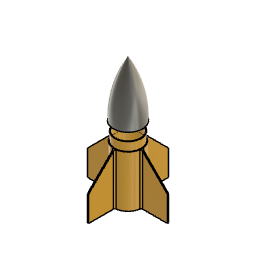
Vlad Rocket 9cone v1 (Autodesk Fusion 360 design; units mm, degrees)
Autodesk Fusion 360 part; units mm, degrees
sketch "Sketch1" plane through (0, 0, 0) normal (0, 0, 1) x (1, 0, 0)
  circle A0 centre (0, 0) radius 12.319
  circle A1 centre (0, 0) radius 11.176
  line L0 (1.016, 25.521) -> (0, 25.521)
  line L1 (-0.508, 25.4) -> (0.508, 25.4)
  line L2 (-0.508, -25.4) -> (-0.508, -12.3085)
  line L3 (0.508, -12.3085) -> (0.508, -25.4)
  line L4 (25.4, 0.508) -> (25.4, -0.508)
  line L5 (0.508, -25.4) -> (-0.508, -25.4)
  line L6 (-25.4, 0.508) -> (-25.4, -0.508)
  line L7 (-0.508, 12.3085) -> (-0.508, 25.4)
  line L8 (0.508, 25.4) -> (0.508, 12.3085)
  line L9 (-25.4, 0.508) -> (-12.3085, 0.508)
  line L10 (-12.3085, -0.508) -> (-25.4, -0.508)
  line L11 (12.3085, 0.508) -> (25.4, 0.508)
  line L12 (25.4, -0.508) -> (12.3085, -0.508)
  dimension "d1" = 24.638
  dimension "d2" = -1.143
  dimension "d8" = 1.016
  constraint coincident A0.centre A1.centre
  constraint horizontal L0
  constraint perpendicular L4 L12
  constraint coincident A0 L7.start
  constraint coincident A0 L8.end
  constraint coincident A0 L9.end
  constraint coincident A0 L10.start
  constraint coincident A0 L12.end
  constraint coincident A0 L11.start
  constraint coincident A0 L3.start
  constraint coincident A0 L2.end
  measures "d1" diameter of A0
  measures "d8" distance of L1.start L1.end
extrude "Extrude1" add sketch "Sketch1" along normal blind 45.72 makes body 1
extrude "Extrude2" add 1 faces at (25.4, 0.1693, 15.24) along direction (1, 0, 0) blind 10.16 on bodies 1 bodies 1
extrude "Extrude3" add 1 faces at (0.1693, -25.4, 15.24) along direction (0, -1, 0) blind 10.16 on bodies 1 bodies 1
extrude "Extrude4" add 1 faces at (-0.1693, 25.4, 15.24) along direction (0, 1, 0) blind 10.16 on bodies 1 bodies 1
extrude "Extrude5" add 1 faces at (-25.4, 0.1693, 15.24) along direction (-1, 0, 0) blind 10.16 on bodies 1 bodies 1
chamfer "Chamfer1" distance 23.241 angle 45 4 edges at (0, 35.56, 45.72) (35.56, 0, 45.72) (0, -35.56, 45.72) (-35.56, 0, 45.72) on bodies 1
sketch "Sketch2" plane through (0, 0, 45.72) normal (0, 0, 1) x (-1, 0, 0)
  line L0 (12.319, -0.508) -> (12.319, 0.508)
  line L1 (12.319, 0.508) -> (12.3085, 0.508)
  arc A0 (12.3085, 0.508) -> (0.508, 12.3085) centre (0, 0) ccw
  line L2 (0.508, 12.3085) -> (0.508, 12.319)
  line L3 (0.508, 12.319) -> (-0.508, 12.319)
  line L4 (-0.508, 12.319) -> (-0.508, 12.3085)
  arc A1 (-0.508, 12.3085) -> (-12.3085, 0.508) centre (0, 0) ccw
  line L5 (-12.3085, 0.508) -> (-12.319, 0.508)
  line L6 (-12.319, 0.508) -> (-12.319, -0.508)
  line L7 (-12.319, -0.508) -> (-12.3085, -0.508)
  arc A2 (-12.3085, -0.508) -> (-0.508, -12.3085) centre (0, 0) ccw
  line L8 (-0.508, -12.3085) -> (-0.508, -12.319)
  line L9 (-0.508, -12.319) -> (0.508, -12.319)
  line L10 (0.508, -12.319) -> (0.508, -12.3085)
  arc A3 (0.508, -12.3085) -> (12.3085, -0.508) centre (0, 0) ccw
  line L11 (12.3085, -0.508) -> (12.319, -0.508)
  circle A4 centre (0, 0) radius 11.176
  circle A5 centre (0, 0) radius 11.176
  circle A6 centre (0, 0) radius 11.7852
  dimension "d22" = 0.6092
  constraint coincident A0.centre A1.centre
extrude "Extrude6" add sketch "Sketch2" along normal blind 7.62 contours A6 bodies 1
fillet "Fillet1" radius 1.27 8 edges at (0.508, -12.3085, 22.86) (12.3085, -0.508, 22.86) (12.3085, 0.508, 22.86) (0.508, 12.3085, 22.86) (-0.508, 12.3085, 22.86) (-12.3085, 0.508, 22.86) (-0.508, -12.3085, 22.86) (-12.3085, -0.508, 22.86) on bodies 1
ref_plane "WorkPlane1" through (24.5161, 0, 22.2834) normal (0, -1, 0) x (1, 0, 0)
sketch "Sketch3" plane through (24.5161, 0, 22.2834) normal (0, -1, 0) x (1, 0, 0)
  arc A0 (-25.4942, 100.8177) -> (-37.7175, 33.3986) centre (183.0643, 28.1876) ccw
  arc A1 (-25.4942, 97.4476) -> (-36.6325, 33.3729) centre (183.0643, 28.1876) ccw
  line L0 (-25.4942, 97.4476) -> (-25.4942, 100.8177)
  line L1 (-36.6325, 33.3729) -> (-37.7175, 33.3986)
  constraint concentric A0 A1
ref_plane "WorkPlane2" through (0, 24.5161, 22.2834) normal (1, 0, 0) x (0, 1, 0)
sketch "Sketch4" plane through (0, 24.5161, 22.2834) normal (1, 0, 0) x (0, 1, 0)
  arc A0 (-10.16, 30.48) -> (-25.4, 88.9) centre (-116.0318, 34.0591) ccw
  line L0 (-12.303, -22.2834) -> (-12.303, 23.4366)
  arc A1 (-11.43, 30.48) -> (-25.4, 87.63) centre (-116.1455, 35.1653) ccw
  line L1 (-10.16, 30.48) -> (-11.43, 30.48)
  line L2 (-25.4, 88.9) -> (-25.4, 87.63)
  constraint tangent A0 A1
  constraint horizontal L1
  constraint perpendicular L1 L2
revolve "Revolve2" add sketch "Sketch4" angle 360 about axis through (0, -0.8839, 111.1834) along (0, 0, -1) separate body makes body 2
scale "Scale1" factor 0.85 about (0, -0.8839, 109.9134) bodies 2
move_body "Align1" bodies 2 to x (1, 0, 0) y (0, 1, 0) z (0, 0, 1) at (0, 0.8839, 0)
